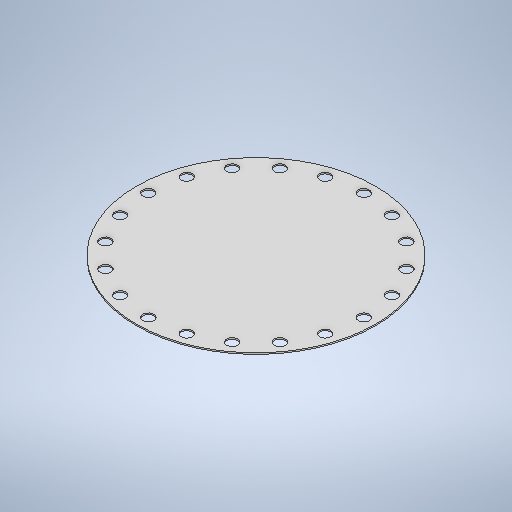
# Autodesk Inventor part: MSC 037 flange cover 500
Saved by Autodesk Inventor 2025 (Build 290162010, 162A)
## iProperties
Created: 2024-06-25
Part Number: MSC 037 flange cover 500
Material: Stainless Steel
Document SubType Name: Sheet Metal
Designer: pokla
Density: 8 g/cm^3
Sheet Metal Rule: AISI304 4mm Die 32
Appearance: Default
Flat Pattern Width: 71 cm
Flat Pattern Length: 71 cm
Flat Pattern Area: 5041 cm^2
Sheet Metal Width: 710,000 mm
Sheet Metal Length: 710,000 mm
Sheet Metal Area: 504100,000 mm^2
Author: pokla
Autodesk Inventor part; units mm, degrees
ref_plane "YZ Plane" through (0, 0, 0) normal (1, 0, 0) x (0, 1, 0)
ref_plane "XZ Plane" through (0, 0, 0) normal (0, 1, 0) x (-1, 0, 0)
ref_plane "XY Plane" through (0, 0, 0) normal (0, 0, 1) x (1, 0, 0)
sketch "Sketch1" plane through (0, 0, 0) normal (0, 0, 1) x (1, 0, 0)
  circle A0 centre (0, 0) radius 355
  dimension "d0" = 710
  measures "d0" diameter of A0
extrude "Plate1" add sketch "Sketch1" against normal blind 4
sketch "Sketch2" plane through (0, 0, 0) normal (0, 0, 1) x (1, 0, 0)
  circle A0 centre (0, 0) radius 320 construction
  circle A1 centre (0, 320) radius 16.5
  dimension "d2" = 640
  dimension "d3" = 33
  constraints: 2 vertical alignment, 1 centre point, 1 coincident, 2 other
  measures "d3" diameter of A1
extrude "Extrusion1" cut sketch "Sketch2" against normal through all
pattern_circular "Circular Pattern1" count 20 over 360 about axis through (0, 0, -10) along (0, 0, 1) of "Extrusion1"
equation "\"d1\" = Thickness"
equation "\"BendReliefWidth\" = Thickness"
equation "\"BendReliefDepth\" = 0.5 * Thickness"
equation "\"CornerReliefSize\" = 4 * Thickness"
equation "\"MinimumRemnant\" = 2 * Thickness"
equation "\"TransitionRadius\" = BendRadius"
equation "\"JacobiRadiusSize\" = BendRadius"
equation "\"GapSize\" = Thickness"
equation "\"Thickness\" = 4"
equation "\"BendRadius\" = 6"
body "Solid1"
